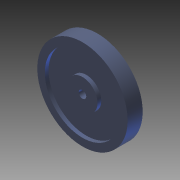
# Autodesk Inventor part: example_wheel_6inch_.5axle
Saved by Autodesk Inventor 2011 (Build 150239000, 239)
## iProperties
Created: 2013-01-17
Part Number: example_wheel_6inch_.5axle
Document SubType Name: Modeling
Designer: Christopher
Density: 1 g/cm^3
Author: Christopher
Autodesk Inventor part; units mm, degrees
ref_plane "YZ Plane" through (0, 0, 0) normal (1, 0, 0) x (0, 1, 0)
ref_plane "XZ Plane" through (0, 0, 0) normal (0, 1, 0) x (-1, 0, 0)
ref_plane "XY Plane" through (0, 0, 0) normal (0, 0, 1) x (1, 0, 0)
sketch "Sketch1" plane through (0, 0, 0) normal (0, 0, 1) x (1, 0, 0)
  circle A0 centre (0, 0) radius 76.2
  circle A1 centre (0, 0) radius 63.5
  circle A2 centre (0, 0) radius 6.35
  circle A3 centre (0, 0) radius 25.4
  dimension "d0" = 152.4
  dimension "d1" = 127
  dimension "d2" = 12.7
  dimension "d3" = 50.8
  constraints: 4 centre point, 4 coincident
  measures "d0" diameter of A0
  measures "d1" diameter of A1
  measures "d2" diameter of A2
  measures "d3" diameter of A3
extrude "Extrusion1" add sketch "Sketch1" along normal mid plane 25.4
extrude "Extrusion2" add sketch "Sketch1" along normal blind 6.35 contours A1
body "Solid1"
